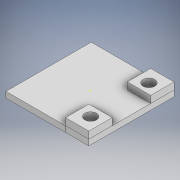
# Autodesk Inventor part: DržačSenzoraUdaljenosti_v.1.0
Saved by Autodesk Inventor 2020 (Build 240168000, 168)
## iProperties
Created: 2020-07-10
Part Number: DržačSenzoraUdaljenosti_v.1.0
Material: Generic
Document SubType Name: Modeling
Designer: Sičaja
Density: 1 g/cm^3
Appearance: Default
Author: Sičaja
Autodesk Inventor part; units mm, degrees
ref_plane "YZ Plane" through (0, 0, 0) normal (1, 0, 0) x (0, 1, 0)
ref_plane "XZ Plane" through (0, 0, 0) normal (0, 1, 0) x (-1, 0, 0)
ref_plane "XY Plane" through (0, 0, 0) normal (0, 0, 1) x (1, 0, 0)
sketch "Sketch1" plane through (0, 0, 0) normal (0, 1, 0) x (-1, 0, 0)
  line L0 (7.1, 7.3) -> (7.1, -7.3)
  line L1 (7.1, -7.3) -> (-7.1, -7.3)
  line L2 (-7.1, -7.3) -> (-7.1, 7.3)
  line L3 (-7.1, 4.95) -> (-7.1, 2.65)
  line L4 (-7.1, 5) -> (-7.1, -5)
  circle A0 centre (-5.1, -5) radius 1
  circle A1 centre (-5.1, 5) radius 1
  line L5 (-7.1, 2.65) -> (-7.1, 4.95)
  line L6 (-7.1, 7.3) -> (7.1, 7.3)
  line L7 (7.1, 7.3) -> (7.1, 0)
  line L8 (-7.1, 4.95) -> (-7.1, 7.3)
  line L9 (-3.1, 7.3) -> (-3.1, -7.3)
  line L10 (-5.1, -3.3) -> (-7.1, -3.3)
  line L11 (-5.1, 3.3) -> (-3.1, 3.3)
  line L12 (-5.1, 3.3) -> (-7.1, 3.3)
  line L13 (-3.1, 3.3) -> (-7.1, 3.3)
  line L14 (-3.1, -3.3) -> (-7.1, -3.3)
  point P0 (0, 0)
  dimension "d4" = 10
  dimension "d6" = 2
  dimension "d7" = 2
  dimension "d8" = 2.3
  dimension "d9" = 14.2
  dimension "d10" = 7.3
  dimension "d14" = 1.7
  dimension "d15" = 1.7
  constraints: 30 end point, 6 point on line, 3 perpendicular, 2 centre point, 2 collinear, 2 vertical, 1 midpoint, 1 parallel
  measures "d4" distance of L4.start L4.end
  measures "d6" diameter of A0
  measures "d7" diameter of A1
  measures "d8" distance of L3.end L3.start
  measures "d9" distance of L0.start L6.start
  measures "d10" distance of L0.start L7.end
  measures "d14" distance of A0.centre L10.start
  measures "d15" distance of A1.centre L11.start
sketch "Sketch2" plane through (0, 0, 0) normal (0, 1, 0) x (-1, 0, 0)
  line L0 (-3.1011, 7.3114) -> (-3.1011, -7.3025)
  line L1 (-3.1011, -7.3025) -> (7.1068, -7.3025)
  line L2 (7.1068, -7.3025) -> (7.1068, 7.3114)
  line L3 (7.1068, 7.3114) -> (-3.1011, 7.3114)
  point P0 (0, 0)
  constraints: 8 end point, 2 perpendicular, 1 horizontal, 1 vertical
extrude "Extrusion1" add sketch "Sketch1" along normal blind 1.2 contours L9 L11 L12 L2 L6 | L1 L2 L10 L14 L9
extrude "Extrusion2" add sketch "Sketch2" against normal blind 1
sketch "Sketch3" plane through (3.1011, 0, 3.3) normal (1, 0, 0) x (0, 0, -1)
  line L0 (10.6025, -1) -> (-4.0114, -1) projected
  line L1 (10.6025, -1) -> (-4.0114, -1)
  line L2 (-4, 0) -> (-4, 1.2) projected
  line L3 (-4.0114, -1) -> (-4, 0)
  line L4 (10.6, 0) -> (6.6, 0) projected
  line L5 (-4, 0) -> (10.6, 0)
  line L6 (10.6025, 0) -> (10.6025, -1) projected
  line L7 (10.6, 0) -> (10.6025, -1)
  point P0 (3.3, 0)
  constraints: 8 end point, 1 collinear, 1 parallel
extrude "Extrusion3" add sketch "Sketch3" along normal blind 4
sketch "Sketch4" plane through (5.1, 0, -5) normal (0, 1, 0) x (1, 0, 0)
  point P0 (-5.1, -5)
sketch "Sketch5" plane through (5.1, 0, -5) normal (0, 1, 0) x (1, 0, 0)
  circle A0 centre (0, 0) radius 1
  point P0 (-5.1, -5)
  dimension "d22" = 2
  constraints: 1 centre point
  measures "d22" diameter of A0
extrude "Extrusion4" cut sketch "Sketch5" against normal blind 1
sketch "Sketch6" plane through (5.1, 0, 5) normal (0, 1, 0) x (1, 0, 0)
  circle A0 centre (0, 0) radius 1
  point P0 (-5.1, 5)
  dimension "d25" = 2
  constraints: 1 centre point
  measures "d25" diameter of A0
extrude "Extrusion5" cut sketch "Sketch6" against normal blind 1
body "Solid1"
